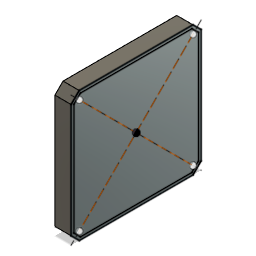
Крышка для крепления под мотор v4 (Autodesk Fusion 360 design; units mm, degrees)
Autodesk Fusion 360 part; units mm, degrees
sketch "Sketch1" plane through (0, 0, 0) normal (1, 0, 0) x (0, 0, -1)
  line L0 (-21, 24) -> (21, 24)
  line L1 (24, 21) -> (24, -21)
  line L2 (21, -24) -> (-21, -24)
  line L3 (-24, -21) -> (-24, 21)
  line L4 (-24, 24) -> (24, -24) construction
  line L5 (24, 24) -> (-24, -24) construction
  line L6 (21, 21) -> (-21, -21) construction
  line L7 (-21, 21) -> (21, -21) construction
  line L8 (-21, 24) -> (-24, 21)
  line L9 (21, 24) -> (24, 21)
  line L10 (-24, -21) -> (-21, -24)
  line L11 (24, -21) -> (21, -24)
  line L12 (23, 20.5858) -> (23, -20.5858)
  line L13 (23, -20.5858) -> (20.5858, -23)
  line L14 (20.5858, -23) -> (-20.5858, -23)
  line L15 (-23, -20.5858) -> (-20.5858, -23)
  line L16 (-23, -20.5858) -> (-23, 20.5858)
  line L17 (-20.5858, 23) -> (-23, 20.5858)
  line L18 (-20.5858, 23) -> (20.5858, 23)
  line L19 (20.5858, 23) -> (23, 20.5858)
  dimension "d1" = 48
  dimension "d2" = 48
  dimension "d3" = 42
  dimension "d4" = 42
  dimension "d5" = 3
  dimension "d6" = 3
  dimension "d7" = 3
  dimension "d8" = 3
  dimension "d9" = 3
  dimension "d10" = 3
  dimension "d11" = 3
  dimension "d12" = 3
  dimension "d13" = 1
  constraint horizontal L0
  constraint perpendicular L0 L1
  constraint parallel L0 L2
  constraint parallel L1 L3
  constraint coincident L4 origin
  constraint coincident L5 origin
  constraint coincident L6 origin
  constraint coincident L7 origin
  constraint coincident L4.start L0
  constraint coincident L4.start L3
  constraint coincident L5.start L0
  constraint coincident L5.start L1
  constraint coincident L5.end L3
  constraint coincident L5.end L2
  constraint coincident L4.end L1
  constraint coincident L4.end L2
  measures "d1" distance of L4.end L5.end
  measures "d2" distance of L5.start L4.end
  measures "d3" distance of L6.end L7.end
  measures "d4" distance of L7.start L6.end
  measures "d5" distance of L4.start L0.start
  measures "d6" distance of L4.start L3.end
  measures "d7" distance of L5.start L0.end
  measures "d8" distance of L5.start L1.start
  measures "d9" distance of L5.end L3.start
  measures "d10" distance of L5.end L2.end
  measures "d11" distance of L4.end L1.end
  measures "d12" distance of L4.end L2.start
extrude "Extrude1" add sketch "Sketch1" against normal blind 6
extrude "Extrude2" add sketch "Sketch1" against normal blind 2 contours L12 L13 L14 L15 L16 L17 L18 L19
equation "d6 = d5"
equation "d8 = d7"
equation "d10 = d9"
equation "d12 = d11"
